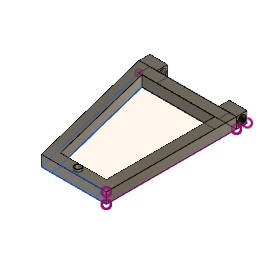
Front Arms (Autodesk Fusion 360 design; units mm, degrees)
Autodesk Fusion 360 part; units mm, degrees
sketch "Top" plane through (0, 0, 0) normal (0, 0, 1) x (1, 0, 0)
  line L0 (0, 0) -> (90, 0)
  line L1 (90, 0) -> (90, -120)
  line L2 (90, -120) -> (30, -120)
  line L3 (0, 0) -> (30, -120)
  line L4 (0, 0) -> (90, 0)
  line L5 (90, 0) -> (90, 10)
  line L6 (90, 10) -> (0, 10)
  line L7 (0, 10) -> (0, 0)
  line L8 (12.8078, -10) -> (80, -10)
  line L9 (80, -10) -> (80, -110)
  line L10 (80, -110) -> (37.8078, -110)
  line L11 (12.8078, -10) -> (37.8078, -110)
  line L12 (39, -110) -> (79, -110)
  line L13 (79, -110) -> (79, -120)
  line L14 (79, -120) -> (39, -120)
  line L15 (39, -120) -> (39, -110)
  line L16 (16.6, 0) -> (73.4, 0)
  line L17 (73.4, 0) -> (73.4, 10)
  line L18 (73.4, 10) -> (16.6, 10)
  line L19 (16.6, 10) -> (16.6, 0)
  dimension "d5" = 90
  dimension "d7" = 60
  dimension "d9" = 10
  dimension "d29" = 40
  dimension "d30" = 10
  dimension "d31" = 1
  dimension "d35" = 10
  dimension "d36" = 56.8
  dimension "d40" = 16.6
  dimension "d41" = 16.6
  constraint coincident L0.start L3.start
  constraint horizontal L0
  constraint perpendicular L0 L1
  constraint perpendicular L1 L2
  constraint horizontal L4
  constraint vertical L5
  constraint horizontal L6
  constraint vertical L7
  constraint horizontal L12
  constraint vertical L13
  constraint horizontal L14
  constraint vertical L15
  constraint coincident L10 L12.start
  constraint horizontal L16
  constraint vertical L17
  constraint horizontal L18
  constraint vertical L19
  constraint coincident L0 L16.start
  measures "d5" distance of L0.start L0.end
  measures "d7" distance of L1.end L2.end
  measures "d9" distance of L0.start L6.end
  measures "d29" distance of L12.start L12.end
  measures "d30" distance of L12.start L14.end
  measures "d31" distance of L9.end L12.end
  measures "d35" distance of L16.start L18.end
  measures "d36" distance of L16.start L16.end
  measures "d40" distance of L7 L19
  measures "d41" distance of L5 L17
extrude "Extrude2" add sketch "Top" along normal blind 10 contours L0 L1 L2 L3 L4 L8 L9 L10 L11 L13 L15 L16 | L2 L10 L12 L13 L14 L15 makes body 1
extrude "Extrude1" add sketch "Top" along normal blind 10 separate body contours L0 L4 L6 L7 L19 | L0 L4 L6 L16 L17 L18 L19 | L0 L4 L5 L6 L17 makes body 2
sketch "Right" plane through (90, 0, 0) normal (1, 0, 0) x (0, 1, 0)
  line L0 (0, 0) -> (10, 0)
  line L1 (10, 0) -> (10, 10)
  line L2 (10, 10) -> (0, 10)
  line L3 (0, 10) -> (0, 0)
  circle A0 centre (5, 5) radius 3.75
  line L4 (0, 0) -> (10, 0)
  line L5 (-120, 0) -> (-120, 10)
  line L6 (0, 0) -> (-120, 0)
  dimension "d15" = 7.5
  dimension "d16" = 5
  dimension "d17" = 5
  measures "d15" diameter of A0
  measures "d16" distance of A0.centre L4
  measures "d17" distance of L1 A0.centre
extrude "Extrude4" cut sketch "Right" against normal blind 190 contours A0 bodies 2
extrude "Extrude3" cut sketch "Right" against normal blind 190 contours A0 bodies 2
extrude "Extrude7" cut sketch "Top" along normal blind 110 contours L0 L4 L6 L16 L17 L18 L19 bodies 2 makes body 3 at (11.0667, 8.7453, 4.8131)
sketch "Sketch3" plane through (0, 0, 10) normal (0, 0, 1) x (-1, 0, 0)
  line L0 (-12.8078, 10) -> (-80, 10)
  line L1 (-80, 10) -> (-80, 110)
  line L2 (-80, 110) -> (-37.8078, 110)
  line L3 (-37.8078, 110) -> (-12.8078, 10)
  line L4 (0, 0) -> (-30, 120)
  line L5 (-30, 120) -> (-90, 120)
  line L6 (-90, 120) -> (-90, 0)
  line L7 (-90, 0) -> (0, 0)
  circle A0 centre (-59, 115) radius 1.5
  circle A1 centre (-59, 115) radius 2.7
  line L8 (-39, 110) -> (-79, 110)
  line L9 (-90, 0) -> (-90, 120)
  line L10 (-79, 110) -> (-79, 120)
  circle A2 centre (-59, 115) radius 3.2
  dimension "d49" = 3
  dimension "d52" = 5.4
  dimension "d55" = 5
  dimension "d57" = 20
  dimension "d58" = 0.5
  constraint concentric A0 A1
  measures "d49" diameter of A0
  measures "d52" diameter of A1
  measures "d55" distance of A0.centre L8
  measures "d57" distance of A0.centre L10
extrude "Extrude10" add sketch "Sketch3" along normal blind 2 contours A2 bodies 1
extrude "Extrude9" cut sketch "Sketch3" against normal blind 4 contours A1 bodies 1
extrude "Extrude8" cut sketch "Sketch3" against normal blind 100 contours A0 bodies 1
equation "wheel_hub_point_width = 60 mm"
equation "chassis_point_full_length = wheel_hub_point_width + ( wheel_hub_point_width / 2 )"
equation "thickness = 10 mm"
equation "length = 100 mm"
equation "d5 = chassis_point_full_length"
equation "d7 = wheel_hub_point_width"
equation "d9 = thickness"
equation "d10 = -thickness"
equation "d11 = thickness"
equation "d13 = thickness"
equation "d15 = 3 * thickness / 4"
equation "d16 = thickness / 2"
equation "d17 = thickness / 2"
equation "d21 = -( chassis_point_full_length + extra )"
equation "d23 = -( chassis_point_full_length + extra )"
equation "extra = 100 mm"
equation "hub_width = 40 mm"
equation "d29 = hub_width"
equation "d30 = thickness"
equation "chassis_point_gap = 56.8 mm"
equation "d35 = thickness"
equation "d36 = chassis_point_gap"
equation "chassis_points_length = 16.6 mm"
equation "d40 = chassis_points_length"
equation "d41 = chassis_points_length"
equation "d42 = thickness + extra"
equation "bearing_682ZZ_outer_radius = 2.7 mm"
equation "bearing_big_distance = hub_width / 2"
equation "bearing_small_distance = thickness / 2"
equation "bearing_682ZZ_inner_radius = 1.5 mm"
equation "bearing_682ZZ_width = 4 mm"
equation "d49 = bearing_682ZZ_inner_radius * 2"
equation "d50 = -extra"
equation "d52 = bearing_682ZZ_outer_radius * 2"
equation "d53 = -bearing_682ZZ_width"
equation "d55 = bearing_small_distance"
equation "d57 = bearing_big_distance"
equation "d58 = bearing_682ZZ_offset"
equation "d59 = bearing_682ZZ_tooth_height"
equation "bearing_682ZZ_tooth_height = 2 mm"
equation "bearing_682ZZ_offset = 0.5 mm"
